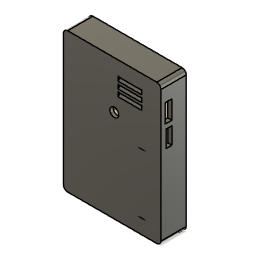
housing Soil_moistV3 v9 (Autodesk Fusion 360 design; units mm, degrees)
Autodesk Fusion 360 part; units mm, degrees
sketch "Sketch1" plane through (0, 0, 0) normal (0, 0, 1) x (1, 0, 0)
  line L0 (53, 0) -> (53, 78)
  line L1 (53, 78) -> (0, 78)
  line L2 (0, 78) -> (0, 0)
  line L3 (55.5, 0) -> (55.5, 78)
  line L4 (53, 80.5) -> (0, 80.5)
  line L5 (-2.5, 78) -> (-2.5, 0)
  arc A0 (0, 80.5) -> (-2.5, 78) centre (0, 78) ccw
  arc A1 (55.5, 78) -> (53, 80.5) centre (53, 78) ccw
  arc A2 (-2.5, 0) -> (0, -2.5) centre (0, 0) ccw
  arc A3 (53, -2.5) -> (55.5, 0) centre (53, 0) ccw
  line L6 (15.75, -2.5) -> (15.75, 0)
  line L7 (37.25, -2.5) -> (37.25, 0)
  line L8 (26.5, 0) -> (26.5, -2.5) construction
  line L9 (0, 0) -> (15.75, 0)
  line L10 (37.25, 0) -> (53, 0)
  line L11 (0, -2.5) -> (15.75, -2.5)
  line L12 (37.25, -2.5) -> (53, -2.5)
  dimension "d1" = 53
  dimension "d2" = 78
  dimension "d4" = 2.5
  dimension "d5" = 21.5
  dimension "d6" = 10.75
  dimension "d7" = 29
  constraint horizontal L9
  constraint vertical L0
  constraint horizontal L1
  constraint vertical L2
  constraint coincident L2.end A2.centre
  constraint tangent L4 A0
  constraint tangent L5 A0
  constraint tangent L3 A1
  constraint tangent L4 A1
  constraint equal A0 A1
  constraint tangent A2 L11
  constraint tangent L5 A2
  constraint equal A0 A2
  constraint tangent A3 L11
  constraint tangent L3 A3
  constraint equal A0 A3
  constraint perpendicular L6 L9
  constraint coincident L7.start L11
  constraint coincident L7.end L9
  constraint perpendicular L7 L9
  constraint collinear L9 L10
  constraint collinear L11 L12
  constraint coincident L8.end L11
  measures "d1" distance of L2.end L0.start
  measures "d2" distance of L2.end L1.end
  measures "d4" radius of A0
  measures "d5" distance of L6 L7
  measures "d6" distance of L7 L8
  measures "d7" distance of L3 L8
sketch "Sketch2" plane through (0, 5.969, 0) normal (0, 1, 0) x (-1, 0, 0)
  line L0 (-53.129, 0) -> (-34.587, 0)
  line L1 (-34.587, 0) -> (-34.587, 1.67)
  line L2 (-34.587, 1.67) -> (-53.129, 1.67)
  line L3 (-53.129, 1.67) -> (-53.129, 0)
  circle A0 centre (-43.858, 0) radius 8.9
  dimension "d12" = 17.8
  constraint midpoint L0 A0.centre
  measures "d12" diameter of A0
extrude "Extrude19" add sketch "Sketch1" along normal blind 10 and the other way blind 5 makes body 1
extrude "Extrude2" add sketch "Sketch2" along normal blind 35.5 separate body contours L0 A0 | L0 L2 A0 | L2 A0 makes body 2
ref_plane "WorkPlane1" through (0, 0, -3) normal (0, 0, 1) x (1, 0, 0)
move_body "Move1" bodies 2 to x (1, 0, 0) y (0, 1, 0) z (0, 0, 1) at (0, 0, 1)
sketch "Back panel" plane through (0, 0, 10) normal (0, 0, 1) x (1, 0, 0)
  line L0 (0, 0) -> (53.3, 0)
  line L1 (53.3, 0) -> (53.3, 77.7)
  line L2 (53.3, 77.7) -> (0, 77.7)
  line L3 (0, 77.7) -> (0, 0)
  line L4 (46.38, 75.3701) -> (49.88, 75.3701)
  line L5 (49.88, 75.3701) -> (49.88, 73.7701)
  line L6 (49.88, 73.7701) -> (46.38, 73.7701)
  line L7 (46.38, 73.7701) -> (46.38, 75.3701)
  line L8 (24.88, 75.3701) -> (28.38, 75.3701)
  line L9 (28.38, 75.3701) -> (28.38, 73.7701)
  line L10 (28.38, 73.7701) -> (24.88, 73.7701)
  line L11 (24.88, 73.7701) -> (24.88, 75.3701)
  line L12 (24.13, 75.9701) -> (29.13, 75.9701)
  line L13 (29.13, 75.9701) -> (29.13, 73.1701)
  line L14 (29.13, 73.1701) -> (24.13, 73.1701)
  line L15 (24.13, 73.1701) -> (24.13, 75.9701)
  line L16 (45.63, 75.9701) -> (50.63, 75.9701)
  line L17 (50.63, 75.9701) -> (50.63, 73.1701)
  line L18 (50.63, 73.1701) -> (45.63, 73.1701)
  line L19 (45.63, 73.1701) -> (45.63, 75.9701)
  line L20 (52.93, 77.45) -> (52.93, 0)
  line L21 (24.93, 46) -> (30.93, 46)
  line L22 (30.93, 46) -> (30.93, 43)
  line L23 (30.93, 43) -> (24.93, 43)
  line L24 (24.93, 43) -> (24.93, 46)
  line L25 (0, 0) -> (0, 77.45)
  line L26 (37.25, 0) -> (37.25, -2.5)
  line L27 (37.25, -2.5) -> (53, -2.5)
  arc A0 (53, -2.5) -> (55.5, 0) centre (53, 0) ccw
  line L28 (55.5, 0) -> (55.5, 78)
  arc A1 (55.5, 78) -> (53, 80.5) centre (53, 78) ccw
  line L29 (53, 80.5) -> (0, 80.5)
  arc A2 (0, 80.5) -> (-2.5, 78) centre (0, 78) ccw
  line L30 (-2.5, 78) -> (-2.5, 0)
  arc A3 (-2.5, 0) -> (0, -2.5) centre (0, 0) ccw
  line L31 (0, -2.5) -> (15.75, -2.5)
  line L32 (15.75, -2.5) -> (15.75, 0)
  line L33 (15.75, 0) -> (0, 0)
  line L34 (0, 0) -> (0, 78)
  line L35 (0, 78) -> (53, 78)
  line L36 (53, 78) -> (53, 0)
  line L37 (53, 0) -> (37.25, 0)
  line L38 (37.25, 0) -> (15.75, 0)
  line L39 (15.75, 0) -> (15.75, -2.5)
  line L40 (15.75, -2.5) -> (37.25, -2.5)
  line L41 (37.25, -2.5) -> (37.25, 0)
  dimension "d16" = 18
  dimension "d17" = 3.5
  dimension "d18" = 3.5
  dimension "d20" = 1.6
  dimension "d21" = 1.6
  dimension "d33" = 2.8
  dimension "d34" = 5
  dimension "d35" = 2.3
  dimension "d36" = 0.75
  dimension "d37" = 0.6
  dimension "d38" = 0.6
  dimension "d41" = 3
  dimension "d42" = 6
  dimension "d43" = 43
  dimension "d45" = 22
  dimension "d193" = 0.75
  constraint horizontal L0
  constraint vertical L1
  constraint horizontal L2
  constraint vertical L3
  constraint coincident L0.start L3.end
  constraint horizontal L4
  constraint vertical L5
  constraint horizontal L6
  constraint vertical L7
  constraint horizontal L8
  constraint vertical L9
  constraint horizontal L10
  constraint vertical L11
  constraint collinear L6 L10
  constraint horizontal L12
  constraint vertical L13
  constraint horizontal L14
  constraint vertical L15
  constraint horizontal L16
  constraint vertical L17
  constraint horizontal L18
  constraint vertical L19
  constraint equal L13 L19
  constraint equal L12 L16
  constraint horizontal L21
  constraint vertical L22
  constraint horizontal L23
  constraint vertical L24
  constraint horizontal L38
  constraint vertical L39
  constraint horizontal L40
  constraint vertical L41
  constraint coincident L31.end L32.start
  constraint coincident L26.start L37.end
  measures "d16" distance of L7 L9
  measures "d17" distance of L4.start L4.end
  measures "d18" distance of L8.start L8.end
  measures "d20" distance of L4.end L5.end
  measures "d21" distance of L8.end L9.end
  measures "d33" distance of L12.start L14.end
  measures "d34" distance of L13.end L14.end
  measures "d35" distance of L17 L20
  measures "d36" distance of L9 L13
  measures "d37" distance of L10 L14
  measures "d38" distance of L6 L18
  measures "d41" distance of L21.end L22.end
  measures "d42" distance of L21.start L21.end
  measures "d43" distance of L0 L23
  measures "d45" distance of L20 L22
  measures "d193" distance of L5 L17
sketch "Sketch4" plane through (0, 41.469, 0) normal (0, 1, 0) x (-1, 0, 0)
  circle A0 centre (-43.858, 1) radius 8.9
  arc A1 (-51.8535, -2.9092) -> (-35.8715, -2.9276) centre (-43.858, 1) ccw
  arc A2 (-52.8008, -2.939) -> (-34.9247, -2.9604) centre (-43.858, 1) ccw
  line L0 (-34.9247, -2.9604) -> (-35.8715, -2.9276)
  line L1 (-51.8535, -2.9092) -> (-52.8008, -2.939)
  line L2 (-44, -2.5) -> (-46.4, -2.5) construction
  constraint coincident A0 A1.start
  constraint coincident A0 A1.end
  constraint coincident A0.centre A1.centre
  constraint horizontal L2
extrude "Extrude4" add sketch "Sketch4" along normal blind -35.5 and the other way blind -7 separate body contours A0 A1 A2 L0 L1 makes body 3
ref_plane "WorkPlane2" through (0, 23.9, 0) normal (0, 1, 0) x (0, 0, 1)
ref_plane "WorkPlane3" through (30, 0, 0) normal (1, 0, 0) x (0, 1, 0)
sketch "USB/switch" plane through (55.5, 0, 0) normal (1, 0, 0) x (0, 0, -1)
  line L0 (1.6, 0) -> (1.6, 77.45)
  line L1 (1.6, 77.45) -> (-8, 77.45)
  line L2 (-8, 77.45) -> (-8, 0)
  line L3 (-8, 0) -> (1.6, 0)
  line L4 (-7.5, 69.95) -> (-3.5, 69.95)
  line L5 (-3.5, 69.95) -> (-3.5, 58.95)
  line L6 (-3.5, 58.95) -> (-7.5, 58.95)
  line L7 (-7.5, 58.95) -> (-7.5, 69.95)
  line L8 (-5.5, 69.95) -> (-5.5, 66.95) construction
  line L9 (-3.2, 77.45) -> (-3.2, 77.6313) construction
  line L10 (-6.95, 56.11) -> (-3.45, 56.11)
  line L11 (-3.45, 56.11) -> (-3.45, 46.11)
  line L12 (-3.45, 46.11) -> (-6.95, 46.11)
  line L13 (-6.95, 46.11) -> (-6.95, 56.11)
  line L14 (-5.2, 56.11) -> (-5.2, 53.11) construction
  line L15 (5, 0) -> (-9, 0)
  line L16 (-9, 0) -> (-9, 77.45)
  line L17 (-9, 77.45) -> (5, 77.45)
  line L18 (5, 77.45) -> (5, 0)
  line L19 (5, 78) -> (-10, 78)
  line L20 (-10, 78) -> (-10, 0)
  line L21 (-10, 0) -> (5, 0)
  line L22 (5, 0) -> (5, 78)
  dimension "d77" = 4
  dimension "d78" = 11
  dimension "d79" = 7.5
  dimension "d80" = 10
  dimension "d81" = 3.5
  dimension "d82" = 2
  dimension "d88" = 2.3
  constraint horizontal L4
  constraint vertical L5
  constraint horizontal L6
  constraint vertical L7
  constraint midpoint L4 L8.start
  constraint perpendicular L4 L8
  constraint midpoint L1 L9.start
  constraint perpendicular L1 L9
  constraint horizontal L10
  constraint vertical L11
  constraint horizontal L12
  constraint vertical L13
  constraint midpoint L10 L14.start
  constraint perpendicular L10 L14
  measures "d77" distance of L4.start L4.end
  measures "d78" distance of L4.start L6.end
  measures "d79" distance of L1 L4
  measures "d80" distance of L10.start L12.end
  measures "d81" distance of L10.start L10.end
  measures "d82" distance of L9 L14
  measures "d88" distance of L8 L9
other "Base Mesh Feature1"
other "Modify1"
sketch "vent" plane through (30, 0, 0) normal (1, 0, 0) x (0, 0, -1)
  line L0 (-13.1067, 68.1626) -> (-11.9577, 67.1984)
  line L1 (-11.9577, 67.1984) -> (-5.675, 74.6858)
  line L2 (-5.675, 74.6858) -> (-6.8241, 75.65)
  line L3 (-13.1067, 68.1626) -> (-6.8241, 75.65)
  line L4 (0, 0) -> (0, 3.2615)
  line L5 (0, 3.2615) -> (0, 20) construction
  line L6 (-8, 77.45) -> (-11, 77.45)
  point P0 (-11, 77.45)
  dimension "d96" = 90
  dimension "d97" = 1.5
  dimension "d98" = 40
  dimension "d99" = 90
  dimension "d102" = 1.8
  constraint perpendicular L0 L1
  constraint coincident L4.start origin
  constraint vertical L4
  constraint parallel L4 L5
  measures "d96" angle of L1 L2
  measures "d97" distance of L1.end L2.end
  measures "d98" angle of L3 L5
  measures "d99" angle of L2 L3
  measures "d102" distance of L2.end L6
extrude "Extrude20" add sketch "Back panel" against normal blind 2 contours L0 L2 L3 L25 L33 L34 L36 L37 L38 | L0 L26 L32 L38 L39 L40 L41 | L2 L34 L35 L36 | L0 L1 L2 L36 | L4 L5 L6 L7 | L8 L9 L10 L11 | L12 L13 L14 L15 | L16 L17 L18 L19 | L21 L22 L23 L24 bodies 1
extrude "Extrude21" add sketch "Back panel" against normal blind 6.2 contours L4 L5 L6 L7 | L8 L9 L10 L11 | L12 L13 L14 L15 | L16 L17 L18 L19 | L21 L22 L23 L24 bodies 1
extrude "Extrude22" add sketch "Back panel" against normal blind 8.5 contours L4 L5 L6 L7 | L8 L9 L10 L11 bodies 1
sketch "Sketch16" plane through (0, 0, 0) normal (0, 0, 1) x (1, 0, 0)
  circle A0 centre (27.7249, 52.3436) radius 2.65
  dimension "d122" = 5.3
  measures "d122" diameter of A0
extrude "Extrude23" cut sketch "Sketch16" along normal blind 14 bodies 1
extrude "Extrude24" cut sketch "vent" along normal blind 14 bodies 1
pattern_linear "R-Pattern3" count 3 spacing 4 along (0, -1, 0) of "Extrude24"
extrude "Extrude25" cut sketch "USB/switch" against normal blind 3 contours L4 L5 L6 L7 | L10 L11 L12 L13 bodies 1
extrude "Extrude27" add sketch "Back panel" against normal blind 5 contours L0 L26 L32 L38 L39 L40 L41 bodies 1
ref_plane "WorkPlane6" through (26.63, 74.5701, -2) normal (0, 0, -1) x (-1, 0, 0)
sketch "cutout" plane through (26.23, 74.32, -2) normal (0, 0, -1) x (1, 0, 0)
  line L0 (27.9256, -4.3244) -> (-27.4785, -4.3244)
  line L1 (-27.4785, -4.3244) -> (-27.4785, 76.8279)
  line L2 (-27.4785, 76.8279) -> (27.9256, 76.8279)
  line L3 (27.9256, 76.8279) -> (27.9256, -4.3244)
  line L4 (26.69, -3.12) -> (-26.211, -3.12)
  line L5 (-26.211, -3.12) -> (-26.211, 74.1)
  line L6 (-26.211, 74.1) -> (26.69, 74.1)
  line L7 (26.69, 74.1) -> (26.69, -3.12)
  line L8 (27.9256, 13.6472) -> (26.69, 13.6472)
  line L9 (26.69, 13.6472) -> (26.69, 23.6472)
  line L10 (26.69, 23.6472) -> (27.9256, 23.6472)
  line L11 (27.9256, 23.6472) -> (27.9256, 13.6472)
  line L12 (-26.211, 13.6472) -> (-27.4785, 13.6472)
  line L13 (-27.4785, 13.6472) -> (-27.4785, 23.6472)
  line L14 (-27.4785, 23.6472) -> (-26.211, 23.6472)
  line L15 (-26.211, 23.6472) -> (-26.211, 13.6472)
  line L16 (-26.211, 0.6472) -> (-27.4785, 0.6472)
  line L17 (-27.4785, 0.6472) -> (-27.4785, 8.6472)
  line L18 (-27.4785, 8.6472) -> (-26.211, 8.6472)
  line L19 (-26.211, 8.6472) -> (-26.211, 0.6472)
  line L20 (27.9256, 0.6472) -> (26.69, 0.6472)
  line L21 (26.69, 0.6472) -> (26.69, 8.6472)
  line L22 (26.69, 8.6472) -> (27.9256, 8.6472)
  line L23 (27.9256, 8.6472) -> (27.9256, 0.6472)
  line L24 (27.9256, 61.8394) -> (26.69, 61.8394)
  line L25 (26.69, 61.8394) -> (26.69, 71.8394)
  line L26 (26.69, 71.8394) -> (27.9256, 71.8394)
  line L27 (27.9256, 71.8394) -> (27.9256, 61.8394)
  line L28 (-26.211, 61.8394) -> (-27.4785, 61.8394)
  line L29 (-27.4785, 61.8394) -> (-27.4785, 71.8394)
  line L30 (-27.4785, 71.8394) -> (-26.211, 71.8394)
  line L31 (-26.211, 71.8394) -> (-26.211, 61.8394)
  line L32 (27.9256, 48.8394) -> (26.69, 48.8394)
  line L33 (26.69, 48.8394) -> (26.69, 56.8394)
  line L34 (26.69, 56.8394) -> (27.9256, 56.8394)
  line L35 (27.9256, 56.8394) -> (27.9256, 48.8394)
  line L36 (-26.211, 48.8394) -> (-27.4785, 48.8394)
  line L37 (-27.4785, 48.8394) -> (-27.4785, 56.8394)
  line L38 (-27.4785, 56.8394) -> (-26.211, 56.8394)
  line L39 (-26.211, 56.8394) -> (-26.211, 48.8394)
  line L40 (-26.211, 74.1) -> (-26.211, 76.8279)
  line L41 (26.69, 74.1) -> (26.69, 76.8279)
  line L42 (-26.211, -3.12) -> (-26.211, -4.3244)
  line L43 (26.69, -3.12) -> (26.69, -4.3244)
  line L44 (-27.1369, 0.6472) -> (-27.1369, 8.6472)
  line L45 (27.6256, 0.6472) -> (27.6256, 8.6472)
  line L46 (27.6256, 48.8394) -> (27.6256, 56.8394)
  line L47 (-27.1369, 48.8394) -> (-27.1369, 56.8394)
  dimension "d152" = 10
  dimension "d153" = 10
  dimension "d154" = 8
  dimension "d155" = 8
  dimension "d156" = 10
  dimension "d157" = 10
  dimension "d158" = 8
  dimension "d159" = 8
  dimension "d160" = 5
  dimension "d161" = 5
  dimension "d194" = 0.3
  dimension "d196" = 0.3415
  constraint horizontal L0
  constraint vertical L1
  constraint horizontal L2
  constraint vertical L3
  constraint horizontal L4
  constraint vertical L5
  constraint horizontal L6
  constraint vertical L7
  constraint horizontal L8
  constraint vertical L9
  constraint horizontal L10
  constraint vertical L11
  constraint coincident L3 L8.start
  constraint horizontal L12
  constraint vertical L13
  constraint horizontal L14
  constraint vertical L15
  constraint coincident L5 L12.start
  constraint collinear L8 L12
  constraint horizontal L16
  constraint vertical L17
  constraint horizontal L18
  constraint vertical L19
  constraint coincident L5 L16.start
  constraint horizontal L20
  constraint vertical L21
  constraint horizontal L22
  constraint vertical L23
  constraint coincident L3 L20.start
  constraint collinear L16 L20
  constraint horizontal L24
  constraint vertical L25
  constraint horizontal L26
  constraint vertical L27
  constraint coincident L3 L24.start
  constraint horizontal L28
  constraint vertical L29
  constraint horizontal L30
  constraint vertical L31
  constraint coincident L5 L28.start
  constraint collinear L24 L28
  constraint horizontal L32
  constraint vertical L33
  constraint horizontal L34
  constraint vertical L35
  constraint coincident L7 L33.end
  constraint coincident L3 L32.start
  constraint horizontal L36
  constraint vertical L37
  constraint horizontal L38
  constraint vertical L39
  constraint coincident L5 L36.start
  constraint collinear L34 L38
  constraint coincident L2 L40.end
  constraint perpendicular L2 L40
  constraint coincident L2 L41.end
  constraint perpendicular L2 L41
  constraint coincident L0 L42.end
  constraint perpendicular L0 L42
  constraint coincident L0 L43.end
  constraint perpendicular L0 L43
  constraint coincident L16 L44.start
  constraint coincident L18 L44.end
  constraint perpendicular L18 L44
  constraint coincident L22 L45.end
  constraint perpendicular L22 L45
  constraint coincident L32 L46.start
  constraint coincident L34 L46.end
  constraint perpendicular L34 L46
  constraint coincident L36 L47.start
  constraint coincident L38 L47.end
  constraint perpendicular L38 L47
  constraint collinear L44 L47
  constraint collinear L45 L46
  measures "d152" distance of L8.start L10.end
  measures "d153" distance of L12.start L14.end
  measures "d154" distance of L16.start L18.end
  measures "d155" distance of L20.start L22.end
  measures "d156" distance of L24.start L26.end
  measures "d157" distance of L28.start L30.end
  measures "d158" distance of L32.start L34.end
  measures "d159" distance of L36.start L38.end
  measures "d160" distance of L12 L18
  measures "d161" distance of L28 L38
  measures "d194" distance of L3 L45
  measures "d196" distance of L1 L44
extrude "Extrude28" cut sketch "cutout" along normal blind 2 contours L0 L3 L7 L20 L43 | L0 L4 L42 L43 | L3 L20 L22 L23 L45 | L0 L1 L5 L16 L42 | L3 L7 L8 L22 | L7 L20 L21 L22 L45 | L3 L7 L8 L9 L10 L11 | L1 L16 L17 L18 L44 | L5 L16 L18 L19 L44 | L3 L7 L10 L32 | L1 L5 L12 L18 | L3 L32 L34 L35 L46 | L1 L5 L12 L13 L14 L15 | L3 L7 L24 L34 | L7 L32 L33 L34 L46 | L1 L5 L14 L36 | L3 L7 L24 L25 L26 L27 | L1 L36 L37 L38 L47 | L5 L36 L38 L39 L47 | L2 L3 L7 L26 L41 | L1 L5 L28 L38 | L1 L5 L28 L29 L30 L31 | L2 L6 L40 L41 | L1 L2 L5 L30 L40 bodies 1
extrude "Extrude29" cut 1 faces at (37.25, -1.6667, -4.6667) along direction (1, 0, 0) up to surface (15.75 mm away) on bodies 1 bodies 1
extrude "Extrude30" cut 1 faces at (15.75, -1.6667, -4.6667) along direction (-1, 0, 0) up to surface (15.75 mm away) on bodies 1 bodies 1
extrude "Extrude34" cut sketch "cutout" along normal up to surface (3 mm away) contours L3 L7 L8 L9 L10 L11 | L1 L5 L12 L13 L14 L15 | L3 L7 L24 L25 L26 L27 | L1 L5 L28 L29 L30 L31 bodies 1
extrude "Extrude35" add sketch "cutout" along normal blind 1.6 separate body contours L0 L4 L42 L43 | L4 L5 L6 L7 L9 L15 L19 L21 L25 L31 L33 L39 | L7 L20 L21 L22 L45 | L5 L16 L18 L19 L44 | L7 L32 L33 L34 L46 | L5 L36 L38 L39 L47 | L2 L3 L7 L26 L41 | L2 L6 L40 L41 | L1 L2 L5 L30 L40 makes body 4
fillet "Fillet4" radius 1 4 edges at (54.1556, -2.5079, -2.8) (-1.2485, -2.5079, -2.8) (0.019, 78.6444, -2.8) (52.92, 78.6444, -2.8) on bodies 4
chamfer "Chamfer2" distance 1.5 distance2 0.5 4 edges at (-0.6242, 50.6728, -5) (-0.6242, 2.4806, -5) (53.5778, 2.4806, -5) (53.5778, 50.6728, -5) measured on face at (17.6667, 78.8333, -5) measured on face at (17.6667, 78.8333, -5) measured on face at (17.6667, 78.8333, -5) measured on face at (17.6667, 78.8333, -5) on bodies 1
sketch "Sketch20" plane through (0, 0, -2) normal (0, 0, 1) x (1, 0, 0)
  arc A0 (-1.2485, -1.5079) -> (-0.2485, -2.5079) centre (-0.2485, -1.5079) ccw
  line L0 (-0.2485, -2.5079) -> (53.1556, -2.5079)
  arc A1 (53.1556, -2.5079) -> (54.1556, -1.5079) centre (53.1556, -1.5079) ccw
  line L1 (54.1556, -1.5079) -> (54.1556, 2.4806)
  line L2 (54.1556, 2.4806) -> (52.92, 2.4806)
  line L3 (52.92, 2.4806) -> (52.92, 17.4806)
  line L4 (52.92, 17.4806) -> (53.8556, 17.4806)
  line L5 (53.8556, 25.4806) -> (52.92, 25.4806)
  line L6 (52.92, 25.4806) -> (52.92, 65.6728)
  line L7 (52.92, 65.6728) -> (53.8556, 65.6728)
  line L8 (53.8556, 73.6728) -> (52.92, 73.6728)
  line L9 (52.92, 73.6728) -> (52.92, 77.6444)
  line L10 (51.92, 78.6444) -> (1.019, 78.6444)
  line L11 (0.019, 77.6444) -> (0.019, 73.6728)
  line L12 (0.019, 73.6728) -> (-0.9069, 73.6728)
  line L13 (-0.9069, 65.6728) -> (0.019, 65.6728)
  line L14 (0.019, 65.6728) -> (0.019, 25.4806)
  line L15 (0.019, 25.4806) -> (-0.9069, 25.4806)
  line L16 (-0.9069, 17.4806) -> (0.019, 17.4806)
  line L17 (0.019, 17.4806) -> (0.019, 2.4806)
  line L18 (0.019, 2.4806) -> (-1.2485, 2.4806)
  line L19 (-1.2485, 2.4806) -> (-1.2485, -1.5079)
  line L20 (15.7543, -2.5079) -> (37.1, -2.5079)
  line L21 (37.1, -2.5079) -> (37.1, -0.5)
  line L22 (37.1, -0.5) -> (15.7543, -0.5)
  line L23 (15.7543, -0.5) -> (15.7543, -2.5079)
  arc A2 (52.92, 77.6444) -> (51.92, 78.6444) centre (51.92, 77.6444) ccw
  arc A3 (1.019, 78.6444) -> (0.019, 77.6444) centre (1.019, 77.6444) ccw
  line L24 (-0.9069, 73.6728) -> (-0.9069, 65.6728)
  line L25 (-0.9069, 25.4806) -> (-0.9069, 17.4806)
  line L26 (53.8556, 17.4806) -> (53.8556, 25.4806)
  line L27 (53.8556, 65.6728) -> (53.8556, 73.6728)
  constraint horizontal L20
  constraint vertical L21
  constraint horizontal L22
  constraint vertical L23
  constraint coincident L0 L20.start
sketch "Sketch21" plane through (30, 0, 0) normal (1, 0, 0) x (0, 0, -1)
  line L0 (1.6433, 76.4069) -> (7.7664, 69.1097)
  line L1 (1.6433, 76.4069) -> (0.4943, 75.4427)
  line L2 (0.4943, 75.4427) -> (6.6173, 68.1455)
  line L3 (7.7664, 69.1097) -> (6.6173, 68.1455)
  line L4 (0, 0) -> (0, 3.2615)
  dimension "d172" = 1.5
  dimension "d173" = 40
  dimension "d174" = 40
  constraint perpendicular L0 L1
  constraint perpendicular L2 L3
  measures "d172" distance of L0.end L2.end
  measures "d173" angle of L2 L4
  measures "d174" angle of L0 L4
extrude "Extrude37" cut sketch "Sketch21" along normal blind 15 bodies 4
pattern_linear "R-Pattern4" count 3 spacing 4 along (0, -1, 0) of "Extrude37"
combine "Combine3" operation cut target body 4 tool bodies 2 keep tools
extrude "Extrude38" cut 1 faces at (41.065, 41.469, -3.0667) along direction (0, 1, 0) blind 7 on bodies 4 bodies 4
sketch "Sketch22" plane through (0, 48.469, 0) normal (0, 1, 0) x (-1, 0, 0)
  line L0 (-51.8535, -2.9092) -> (-52.8008, -2.939)
  arc A0 (-52.8008, -2.939) -> (-34.9247, -2.9604) centre (-43.858, 1) ccw
  line L1 (-34.9247, -2.9604) -> (-35.8715, -2.9276)
  arc A1 (-51.8535, -2.9092) -> (-35.8715, -2.9276) centre (-43.858, 1) ccw
  line L2 (-52.8008, -2.939) -> (-35.3981, -2.944)
  arc A2 (-52.8008, -2.939) -> (-35.3981, -2.944) centre (-44.0984, 0.5842) ccw
  constraint coincident L0.end A0.start
  constraint midpoint L1 L2.end
revolve "Revolve2" add 1 faces at (43.8687, 48.469, -8.1742) angle 80 about axis through (35.4789, 48.469, -2) along (1, 0, 0) on bodies 3 bodies 3 4
sketch "Sketch23" plane through (0, 5.969, 0) normal (0, -1, 0) x (1, 0, 0)
  line L0 (52.4794, -3.6) -> (51.4771, -3.6)
  arc A0 (36.2389, -3.6) -> (51.4771, -3.6) centre (43.858, 1) ccw
  line L1 (36.2389, -3.6) -> (35.2366, -3.6)
  arc A1 (35.2366, -3.6) -> (52.4794, -3.6) centre (43.858, 1) ccw
  line L2 (51.4771, -3.6) -> (36.2389, -3.6)
  constraint coincident L0.end A0.end
  constraint coincident A0.start L1.start
revolve "Revolve3" add sketch "Sketch23" angle 90 about axis through (51.4771, 5.969, -3.6) along (-1, 0, 0) contours L0 A0 L1 A1 bodies 3
combine "Combine4" operation cut target body 1 tool bodies 2 keep tools
extrude "Extrude42" cut 1 faces at (46.3977, 5.969, -2.5333) along direction (0, -1, 0) blind 1.5 on bodies 3 bodies 3
extrude "Extrude43" cut 1 faces at (46.3977, 48.469, -2.5333) along direction (0, 1, 0) blind 2.5 on bodies 3 bodies 3
extrude "Extrude39" [suppressed]
extrude "Extrude40" [suppressed]
extrude "Extrude41" [suppressed]
named bodies: "Batterie", "capac baterie", "carcasa"
